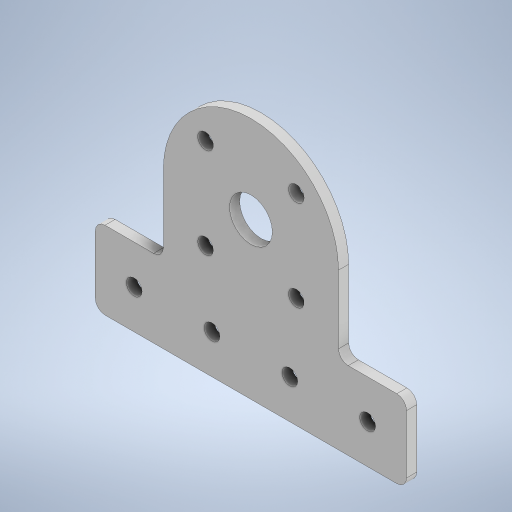
# Autodesk Inventor part: ArmPlateBase V2
Saved by Autodesk Inventor 2024 (Build 280153000, 153)
## iProperties
Created: 2024-01-11
Part Number: ArmPlateBase V2
Material: Generic
Document SubType Name: Modeling
Designer: megan
Density: 1 g/cm^3
Appearance: Default
Author: megan
Autodesk Inventor part; units mm, degrees
ref_plane "YZ Plane" through (0, 0, 0) normal (1, 0, 0) x (0, 1, 0)
ref_plane "XZ Plane" through (0, 0, 0) normal (0, 1, 0) x (-1, 0, 0)
ref_plane "XY Plane" through (0, 0, 0) normal (0, 0, 1) x (1, 0, 0)
sketch "Sketch1" plane through (0, 0, 0) normal (0, 0, 1) x (1, 0, 0)
  arc A0 (28.575, 0) -> (-28.575, 0) centre (0, 0) ccw
  circle A1 centre (0, 0) radius 7
  line L0 (-19, -50.8) -> (19, -50.8)
  line L1 (28.575, -25.4) -> (28.575, 0)
  line L2 (-28.575, 0) -> (-28.575, -25.4)
  line L3 (0, -66.675) -> (0, 44.45) projected
  circle A2 centre (-12.7, -38.1) radius 2.5781
  circle A3 centre (12.7, -38.1) radius 2.5781
  line L4 (-19, -50.8) -> (-50.8, -50.8)
  line L5 (-50.8, -50.8) -> (-50.8, -25.4)
  line L6 (50.8, -25.4) -> (50.8, -50.8)
  line L7 (50.8, -50.8) -> (-50.8, -50.8)
  line L8 (-50.8, -25.4) -> (-28.575, -25.4)
  line L9 (28.575, -25.4) -> (50.8, -25.4)
  circle A4 centre (-38.1, -38.1) radius 2.5781
  circle A5 centre (38.1, -38.1) radius 2.5781
  dimension "d1" = 14
  dimension "d10" = 5.1562
  dimension "d11" = 5.1562
  dimension "d12" = 12.7
  dimension "d13" = 12.7
  dimension "d14" = 12.7
  dimension "d15" = 12.7
  dimension "d16" = 50.8
  dimension "d17" = 25.4
  dimension "d18" = 101.6
  dimension "d19" = 50.8
  dimension "d20" = 25.4
  dimension "d21" = 25.4
  dimension "d25" = 28.575
  dimension "d26" = 25.4
  constraints: 18 end point, 7 perpendicular, 6 centre point, 2 coincident, 2 equal radius, 2 parallel, 2 point on circle, 1 horizontal, 1 point on line, 1 tangent
  measures "d1" diameter of A1
  measures "d10" diameter of A2
  measures "d11" diameter of A3
  measures "d12" distance from line of L0 A2.centre
  measures "d13" distance from line of L0 A3.centre
  measures "d14" distance from line of L3 A2.centre
  measures "d15" distance from line of L3 A3.centre
  measures "d16" distance from line of L0 point (0, 0)
  measures "d17" distance of L4.end L5.end
  measures "d18" distance between parallel lines of L6 L5
  measures "d19" distance between parallel lines of L5 L3
  measures "d20" distance of A2.centre A4.centre
  measures "d21" distance of A5.centre A3.centre
  measures "d25" radius of A0
  measures "d26" distance from line of L8 A0.centre
extrude "Extrusion1" add sketch "Sketch1" along normal blind 3.302 contours L1 L9 L6 L7 L0 L3 A1 A0 | L3 A1 L0 L4 L5 L8 L2 A0
fillet "Fillet1" radius 3.175 6 edges at (28.575, -25.4, 1.651) (-28.575, -25.4, 1.651) (-50.8, -25.4, 1.651) (-50.8, -50.8, 1.651) (50.8, -25.4, 1.651) (50.8, -50.8, 1.651)
sketch "Sketch2" plane through (0, 0, 3.302) normal (0, 0, 1) x (1, 0, 0)
  circle A0 centre (0, 0) radius 12
  circle A1 centre (0, 0) radius 20.955
  circle A2 centre (0, 0) radius 7 projected
  line L0 (0, 0) -> (14.8174, 14.8174)
  line L1 (0, 0) -> (12, 0) construction
  dimension "d27" = 24
  dimension "d28" = 41.91
  dimension "d29" = 45
  constraints: 4 end point, 2 coincident, 1 horizontal, 1 horizontal alignment, 5 other
  measures "d29" angle of L1 L0
hole "Hole1" at (14.8174, 14.8174, 3.302) direction (0, 0, -1) diameter 5.1054 depth 16.256 tip angle 118 clearance for "Flat Head Machine Screw (82)" size "#10" standard "Ansi Unified Screw Threads"
pattern_circular "Circular Pattern1" count 4 over 360 about axis through (0, 0, 0) along (0, 0, 1) of "Hole1"
equation "\"d19\" = 0.5 * d18"
body "Solid1"
